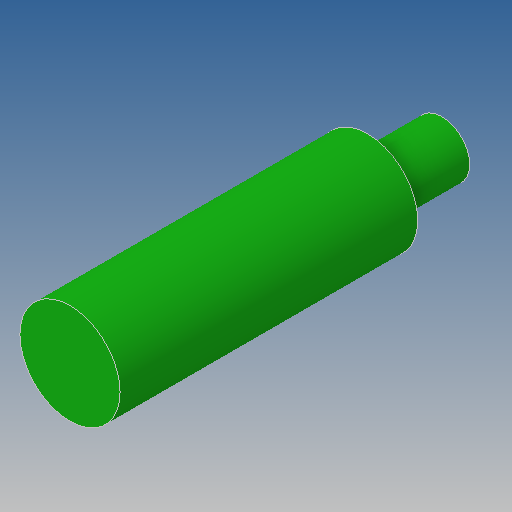
# Autodesk Inventor part: Handle
Saved by Autodesk Inventor 2018 (Build 220112000, 112)
## iProperties
Created: 2022-02-21
Part Number: Handle
Material: Generic
Document SubType Name: Modeling
Designer: Nathann
Density: 1 g/cm^3
Appearance: Default
Author: Nathann
Autodesk Inventor part; units mm, degrees
ref_plane "YZ Plane" through (0, 0, 0) normal (1, 0, 0) x (0, 1, 0)
ref_plane "XZ Plane" through (0, 0, 0) normal (0, 1, 0) x (-1, 0, 0)
ref_plane "XY Plane" through (0, 0, 0) normal (0, 0, 1) x (1, 0, 0)
sketch "Sketch1" plane through (0, 0, 0) normal (0, 0, 1) x (1, 0, 0)
  circle A0 centre (50.6547, -20.9505) radius 7.452 projected
  circle A1 centre (50.6547, -20.9505) radius 7.452
  point P0 (0, 0)
  constraints: 1 centre point, 1 coincident, 1 concentric
extrude "Extrusion1" add sketch "Sketch1" along normal mid plane 20
sketch "Sketch2" plane through (50.6547, -20.9505, 10) normal (0, 0, 1) x (1, 0, 0)
  circle A0 centre (0, 0) radius 13.4659
  point P0 (-50.6547, 20.9505)
  constraints: 1 centre point
extrude "Extrusion2" add sketch "Sketch2" along normal blind 80
body "Solid1"
